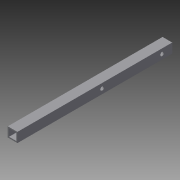
# Autodesk Inventor part: custom box alluminum 8in
Saved by Autodesk Inventor 2013 (Build 170138000, 138)
## iProperties
Created: 2013-12-23
Part Number: custom box alluminum 8in
Material: Generic
Document SubType Name: Modeling
Designer: kahohbein
Density: 1 g/cm^3
Author: kahohbein
Autodesk Inventor part; units mm, degrees
ref_plane "YZ Plane" through (0, 0, 0) normal (1, 0, 0) x (0, 1, 0)
ref_plane "XZ Plane" through (0, 0, 0) normal (0, 1, 0) x (-1, 0, 0)
ref_plane "XY Plane" through (0, 0, 0) normal (0, 0, 1) x (1, 0, 0)
sketch "Sketch1" plane through (0, 0, 0) normal (0, 0, 1) x (1, 0, 0)
  line L0 (-6.35, -6.35) -> (6.35, -6.35)
  line L1 (6.35, -6.35) -> (6.35, 6.35)
  line L2 (6.35, 6.35) -> (-6.35, 6.35)
  line L3 (-6.35, 6.35) -> (-6.35, -6.35)
  line L4 (-6.35, -6.35) -> (6.35, 6.35) construction
  line L5 (6.35, -6.35) -> (-6.35, 6.35) construction
  line L6 (-4.7625, -4.7625) -> (4.7625, -4.7625)
  line L7 (4.7625, -4.7625) -> (4.7625, 4.7625)
  line L8 (4.7625, 4.7625) -> (-4.7625, 4.7625)
  line L9 (-4.7625, 4.7625) -> (-4.7625, -4.7625)
  line L10 (-4.7625, -4.7625) -> (4.7625, 4.7625) construction
  line L11 (4.7625, -4.7625) -> (-4.7625, 4.7625) construction
  point P0 (0, 0)
  point P1 (0, 0)
  dimension "d0" = 12.7
  dimension "d1" = 12.7
  dimension "d2" = 9.525
  dimension "d3" = 9.525
  constraints: 24 end point, 4 midpoint, 4 parallel, 2 horizontal, 2 perpendicular
  measures "d0" distance of L2.end L1.end
  measures "d1" distance of L1.end L0.end
  measures "d2" distance of L8.end L7.end
  measures "d3" distance of L7.end L6.end
extrude "Extrusion1" add sketch "Sketch1" along normal blind 203.2
sketch "Sketch2" plane through (6.35, -6.35, 0) normal (1, 0, 0) x (0, 0, -1)
  line L0 (0, 0) -> (-203.2, 0) projected
  circle A0 centre (-13.3193, 6.35) radius 2.413
  circle A1 centre (-91.9323, 6.35) radius 2.413
  line L1 (-89.5193, 6.35) -> (-13.3193, 6.35)
  point P0 (0, 6.35)
  dimension "d7" = 4.826
  dimension "d6" = 4.826
  dimension "d8" = 76.2
  constraints: 2 end point, 1 centre point, 1 horizontal alignment, 1 parallel, 2 other
  measures "d6" diameter of A0
  measures "d8" distance of L1.start L1.end
extrude "Extrusion2" cut sketch "Sketch2" against normal blind 203.2
body "Solid1"
